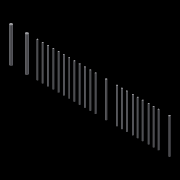
# Autodesk Inventor part: 3d_LM-Welding_Tooling - Wire
Saved by Autodesk Inventor 2018.3 (Build 223284000, 284)
## iProperties
Created: 2026-01-21
Part Number: 3d_LM-Welding_Tooling - Wire
Material: Genérico
Document SubType Name: Modeling
Designer: aca6
Density: 1 g/cm^3
Appearance: Valor por defecto
Author: aca6
Autodesk Inventor part; units mm, degrees
ref_plane "YZ Plane" through (0, 0, 0) normal (1, 0, 0) x (0, 1, 0)
ref_plane "XZ Plane" through (0, 0, 0) normal (0, 1, 0) x (-1, 0, 0)
ref_plane "XY Plane" through (0, 0, 0) normal (0, 0, 1) x (1, 0, 0)
sketch "Sketch1" plane through (0, 0, 0) normal (0, 0, 1) x (1, 0, 0)
  line L0 (0, 0) -> (0, 3.9873) construction
  line L1 (0, 0) -> (2.2526, 0) construction
  circle A0 centre (22.5, 0) radius 0.255
  circle A1 centre (19.4, 0) radius 0.2025
  circle A2 centre (18, 0) radius 0.2025
  circle A3 centre (16.6, 0) radius 0.2025
  circle A4 centre (14.9, 0) radius 0.2025
  circle A5 centre (13.5, 0) radius 0.2025
  circle A6 centre (12.1, 0) radius 0.2025
  circle A7 centre (10.4, 0) radius 0.2025
  circle A8 centre (9, 0) radius 0.2025
  circle A9 centre (7.6, 0) radius 0.2025
  circle A10 centre (4.5, 0) radius 0.255
  circle A11 centre (1.5, 0) radius 0.2025
  circle A12 centre (0, 0) radius 0.2025
  circle A13 centre (-1.5, 0) radius 0.2025
  circle A14 centre (-3, 0) radius 0.2025
  circle A15 centre (-4.5, 0) radius 0.2025
  circle A16 centre (-6, 0) radius 0.2025
  circle A17 centre (-7.5, 0) radius 0.2025
  circle A18 centre (-9, 0) radius 0.2025
  circle A19 centre (-10.5, 0) radius 0.2025
  circle A20 centre (-12, 0) radius 0.2025
  circle A21 centre (-13.5, 0) radius 0.2025
  circle A22 centre (-15, 0) radius 0.2025
  circle A23 centre (-18, 0) radius 0.405
  circle A24 centre (-22.5, 0) radius 0.405
  dimension "d1" = 0.51
  dimension "d2" = 0.405
  dimension "d3" = 0.405
  dimension "d4" = 0.405
  dimension "d5" = 0.405
  dimension "d6" = 0.405
  dimension "d7" = 0.405
  dimension "d8" = 0.405
  dimension "d9" = 0.405
  dimension "d10" = 0.405
  dimension "d11" = 0.51
  dimension "d12" = 0.405
  dimension "d13" = 0.405
  dimension "d14" = 0.405
  dimension "d15" = 0.405
  dimension "d16" = 0.405
  dimension "d17" = 0.405
  dimension "d18" = 0.405
  dimension "d19" = 0.405
  dimension "d20" = 0.405
  dimension "d21" = 0.405
  dimension "d22" = 0.405
  dimension "d23" = 0.405
  dimension "d24" = 0.81
  dimension "d25" = 0.81
  dimension "d26" = 3.1
  dimension "d27" = 1.4
  dimension "d28" = 1.4
  dimension "d29" = 1.7
  dimension "d30" = 1.4
  dimension "d31" = 1.4
  dimension "d32" = 1.7
  dimension "d33" = 1.4
  dimension "d34" = 1.4
  dimension "d35" = 3.1
  dimension "d36" = 3
  dimension "d37" = 1.5
  dimension "d38" = 1.5
  dimension "d39" = 1.5
  dimension "d40" = 1.5
  dimension "d41" = 1.5
  dimension "d42" = 1.5
  dimension "d43" = 1.5
  dimension "d44" = 1.5
  dimension "d45" = 1.5
  dimension "d46" = 1.5
  dimension "d47" = 1.5
  dimension "d48" = 3
  dimension "d49" = 4.5
  constraints: 25 centre point, 4 end point, 2 horizontal, 2 vertical, 1 coincident, 1 point on line, 3 other
  measures "d1" diameter of A0
  measures "d2" diameter of A1
  measures "d3" diameter of A2
  measures "d4" diameter of A3
  measures "d5" diameter of A4
  measures "d6" diameter of A5
  measures "d7" diameter of A6
  measures "d8" diameter of A7
  measures "d9" diameter of A8
  measures "d10" diameter of A9
  measures "d11" diameter of A10
  measures "d12" diameter of A11
  measures "d13" diameter of A12
  measures "d14" diameter of A13
  measures "d15" diameter of A14
  measures "d16" diameter of A15
  measures "d17" diameter of A16
  measures "d18" diameter of A17
  measures "d19" diameter of A18
  measures "d20" diameter of A19
  measures "d21" diameter of A20
  measures "d22" diameter of A21
  measures "d23" diameter of A22
  measures "d24" diameter of A23
  measures "d25" diameter of A24
  measures "d26" distance of A1.centre A0.centre
  measures "d27" distance of A2.centre A1.centre
  measures "d28" distance of A3.centre A2.centre
  measures "d29" distance of A4.centre A3.centre
  measures "d30" distance of A5.centre A4.centre
  measures "d31" distance of A6.centre A5.centre
  measures "d32" distance of A7.centre A6.centre
  measures "d33" distance of A8.centre A7.centre
  measures "d34" distance of A8.centre A9.centre
  measures "d35" distance of A10.centre A9.centre
  measures "d36" distance of A11.centre A10.centre
  measures "d37" distance of L0.start A11.centre
  measures "d38" distance of A13.centre L0.start
  measures "d39" distance of A14.centre A13.centre
  measures "d40" distance of A15.centre A14.centre
  measures "d41" distance of A15.centre A16.centre
  measures "d42" distance of A16.centre A17.centre
  measures "d43" distance of A18.centre A17.centre
  measures "d44" distance of A18.centre A19.centre
  measures "d45" distance of A19.centre A20.centre
  measures "d46" distance of A20.centre A21.centre
  measures "d47" distance of A21.centre A22.centre
  measures "d48" distance of A22.centre A23.centre
  measures "d49" distance of A23.centre A24.centre
extrude "Extrusion1" add sketch "Sketch1" along normal blind 10
body "Solid1"
